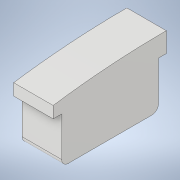
# Autodesk Inventor part: canopy
Saved by Autodesk Inventor 2020 (Build 240168000, 168)
## iProperties
Part Number: canopy
Material: PC/ABS-Kunststoff
Document SubType Name: Modeling
Designer: Admin
Mass: 1220.8 g
Surface Area: 691.534 cm^2
Volume: 1070.88 cm^3
Density: 0.357273 g/cm^3
Appearance: Glatt - Weiß
Gewicht: 1,221 kg
G_L: 0
G_H: 0
G_B: 0
InventorVersion: 2019.4
VAULT_Status: in Bearbeitung
Revision: -
Max. Breite: 0
Max. Höhe: 0
Max. Länge: 0
Max. Abmessungen: 0 x 0 x 0
Author: Admin
Autodesk Inventor part; units mm, degrees
note: some values were not read from the file. Left out: dimensions or parameters whose unit could not be read.
ref_plane "YZ Plane" through (0, 0, 0) normal (1, 0, 0) x (0, 1, 0)
ref_plane "XZ Plane" through (0, 0, 0) normal (0, 1, 0) x (-1, 0, 0)
ref_plane "XY Plane" through (0, 0, 0) normal (0, 0, 1) x (1, 0, 0)
sketch "Skizze1" plane through (0, 0, 0) normal (0, 0, 1) x (1, 0, 0)
  line L0 (-30, -80) -> (30, -80)
  line L1 (30, -80) -> (30, 80)
  line L2 (30, 80) -> (-30, 80)
  line L3 (-30, 80) -> (-30, -80)
  line L4 (-30, -80) -> (30, 80) construction
  line L5 (30, -80) -> (-30, 80) construction
  point P0 (0, 0)
  dimension "d0" = 60
  dimension "d1" = 160
  constraints: 12 end point, 2 midpoint, 2 parallel, 1 horizontal, 1 perpendicular
  measures "d0" distance of L2.end L1.end
  measures "d1" distance of L1.end L0.end
extrude "Extrusion1" add sketch "Skizze1" along normal blind 100
sketch "Skizze5" plane through (30, -80, 0) normal (1, 0, 0) x (0, 0, -1)
  line L0 (0, 0) -> (-70, 0)
  line L1 (-70, 0) -> (-70, 13)
  line L2 (-70, 13) -> (0, 13)
  line L3 (0, 13) -> (0, 0)
  point P0 (0, 80)
  dimension "d15" = 70
  dimension "d16" = 13
  constraints: 8 end point, 2 parallel, 1 horizontal, 1 perpendicular
  measures "d15" distance of L1.end L2.end
  measures "d16" distance of L0.end L1.end
extrude "Extrusion5" cut sketch "Skizze5" against normal through all
sketch "Skizze6" plane through (30, 80, 100) normal (1, 0, 0) x (0, 0, -1)
  line L0 (100, 0) -> (0, 0) projected
  line L1 (0, 0) -> (30, 0)
  line L2 (30, 0) -> (30, 12)
  line L3 (30, 12) -> (0, 12)
  line L4 (0, 12) -> (0, 0)
  point P0 (100, -80)
  point P1 (30, 0)
  dimension "d24" = 30
  dimension "d25" = 12
  constraints: 8 end point, 2 parallel, 1 horizontal, 1 perpendicular
  measures "d24" distance of L3.end L2.end
  measures "d25" distance of L2.end L1.end
extrude "Extrusion6" add sketch "Skizze6" against normal up to surface (60 mm away)
fillet "Rundung1" radius 10 2 edges at (0, -67, 0) (0, 80, 0)
sketch "Skizze7" plane through (30, -80, 70) normal (1, 0, 0) x (0, 0, -1)
  line L0 (-30, 0) -> (-17.65, 0)
  line L1 (0, 0) -> (-30, 0) projected
  line L2 (-30, 0) -> (-30, 172) projected
  line L3 (-30, 0) -> (-30, 172)
  spline S0 degree 2 poles (-30, 172) (-30, 85.6679) (-17.65, 0) knots 0 0 0 1 1 1
  point P0 (70, 80)
  dimension "d27" = 12.35
  constraints: 4 end point, 2 vertical, 1 point on line, 2 other
  measures "d27" distance of L0.start L0.end
extrude "Extrusion7" cut sketch "Skizze7" against normal up to next
equation "\"G_L\" = 0"
equation "\"G_H\" = 0"
equation "\"G_B\" = 0"
